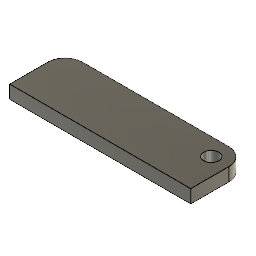
3.5 mirror (Autodesk Fusion 360 design; units mm, degrees)
Autodesk Fusion 360 part; units mm, degrees
sketch "Sketch1" plane through (0, 0, 0) normal (0, 0, 1) x (1, 0, 0)
  line L0 (0, 0) -> (42.3969, 0)
  line L1 (42.3969, 0) -> (42.3969, 17.8119)
  line L2 (34.1572, 26.0516) -> (0, 26.0516)
  line L3 (-42.3969, 0) -> (-42.3969, 17.8119)
  line L4 (-34.1572, 26.0516) -> (0, 26.0516)
  line L5 (0, 0) -> (-42.3969, 0)
  arc A0 (-34.1572, 26.0516) -> (-42.3969, 17.8119) centre (-34.1572, 17.8119) ccw
  arc A1 (42.3969, 17.8119) -> (34.1572, 26.0516) centre (34.1572, 17.8119) ccw
  circle A2 centre (34.1572, 17.8119) radius 3.5265
  dimension "d1" = 8.2397
  measures "d1" radius of A0
extrude "Extrude1" add sketch "Sketch1" along normal blind 6.276
